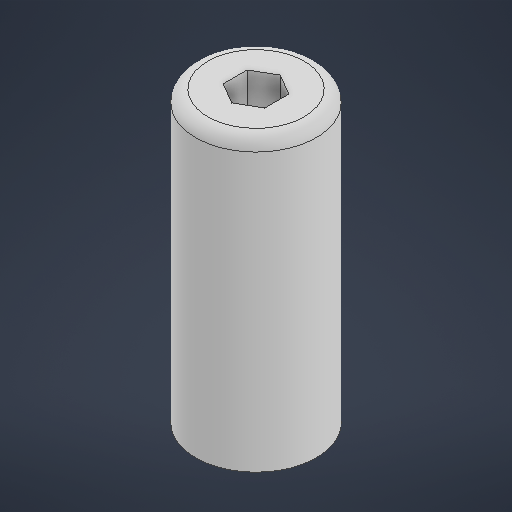
# Autodesk Inventor part: 5mm Screw
Saved by Autodesk Inventor 2026.2 (Build 302298000, 298)
## iProperties
Created: 2025-12-10
Part Number: 5mm Screw
Material: Generic
Document SubType Name: Modeling
Designer: Thoma
Density: 1 g/cm^3
Appearance: Default
Author: Thoma
Autodesk Inventor part; units mm, degrees
ref_plane "YZ Plane" through (0, 0, 0) normal (1, 0, 0) x (0, 1, 0)
ref_plane "XZ Plane" through (0, 0, 0) normal (0, 1, 0) x (-1, 0, 0)
ref_plane "XY Plane" through (0, 0, 0) normal (0, 0, 1) x (1, 0, 0)
sketch "Sketch1" plane through (0, 0, 0) normal (0, 1, 0) x (-1, 0, 0)
  circle A0 centre (0, 0) radius 2.5
  dimension "d0" = 5
  constraints: 1 centre point, 1 coincident
  measures "d0" diameter of A0
extrude "Extrusion1" add sketch "Sketch1" along normal blind 12
fillet "Fillet1" radius 0.5 1 edges at (2.5, 12, 0)
sketch "Sketch2" plane through (0, 12, 0) normal (0, 1, 0) x (1, 0, 0)
  line L0 (0, 1) -> (0.866, 0.5)
  line L1 (0.866, 0.5) -> (0.866, -0.5)
  line L2 (0.866, -0.5) -> (0, -1)
  line L3 (0, -1) -> (-0.866, -0.5)
  line L4 (-0.866, -0.5) -> (-0.866, 0.5)
  line L5 (-0.866, 0.5) -> (0, 1)
  point P0 (0, 0)
  point P1 (0, 0)
  dimension "d4" = 1
  constraints: 12 end point, 1 coincident, 13 other
  measures "d4" distance of L4.end L3.end
extrude "Extrusion2" cut sketch "Sketch2" against normal blind 2
body "Solid1"
